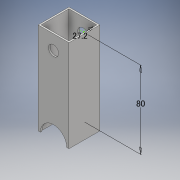
# Autodesk Inventor part: 軸受上用
Saved by Autodesk Inventor 2018 (Build 220112000, 112)
## iProperties
Created: 2017-09-13
Part Number: 軸受上用
Material: 一般
Document SubType Name: Modeling
Designer: mura5
Density: 1 g/cm^3
Appearance: 既定
Author: mura5
Autodesk Inventor part; units mm, degrees
ref_plane "YZ Plane" through (0, 0, 0) normal (1, 0, 0) x (0, 1, 0)
ref_plane "XZ Plane" through (0, 0, 0) normal (0, 1, 0) x (-1, 0, 0)
ref_plane "XY Plane" through (0, 0, 0) normal (0, 0, 1) x (1, 0, 0)
sketch "スケッチ1" plane through (0, 0, 0) normal (0, 0, 1) x (1, 0, 0)
  line L0 (-16, -16) -> (16, -16)
  line L1 (16, -16) -> (16, 16)
  line L2 (16, 16) -> (-16, 16)
  line L3 (-16, 16) -> (-16, -16)
  line L4 (-16, -16) -> (16, 16) construction
  line L5 (16, -16) -> (-16, 16) construction
  line L6 (-14.4, 14.4) -> (14.4, 14.4)
  line L7 (14.4, 14.4) -> (14.4, -14.4)
  line L8 (14.4, -14.4) -> (-14.4, -14.4)
  line L9 (-14.4, -14.4) -> (-14.4, 14.4)
  point P0 (0, 0)
  dimension "d0" = 32
  dimension "d1" = 32
  dimension "d2" = 1.6
  constraints: 20 end point, 4 parallel, 2 midpoint, 2 perpendicular, 1 horizontal, 3 other
  measures "d0" distance of L2.end L1.end
  measures "d1" distance of L1.end L0.end
  measures "d2" distance between parallel lines of L2 L6
extrude "押し出し1" add sketch "スケッチ1" along normal blind 95
sketch "スケッチ2" plane through (-16, 16, 0) normal (0, 1, 0) x (1, 0, 0)
  circle A0 centre (16, 0) radius 13.6
  dimension "d5" = 27.2
  constraints: 1 centre point, 1 coincident
  measures "d5" diameter of A0
extrude "押し出し2" cut sketch "スケッチ2" against normal blind 32
sketch "スケッチ3" plane through (-16, 16, 95) normal (0, 1, 0) x (1, 0, 0)
  line L0 (32, 0) -> (0, 0) projected
  point P0 (16, 95)
  point P1 (16, 15)
  dimension "d16" = 80
  measures "d16" distance of point (16, 15) point (16, 95)
hole "穴1" at (0, 16, 80) direction (0, -1, 0) diameter 10.5 end through all
sketch "スケッチ4" plane through (-16, 16, 95) normal (0, 1, 0) x (1, 0, 0)
  circle A0 centre (16, 15) radius 13.6
  point P0 (16, 95)
  dimension "d17" = 80
  dimension "d18" = 27.2
  constraints: 1 centre point, 1 coincident
  measures "d17" distance of point (16, 95) point (16, 15)
  measures "d18" diameter of A0
